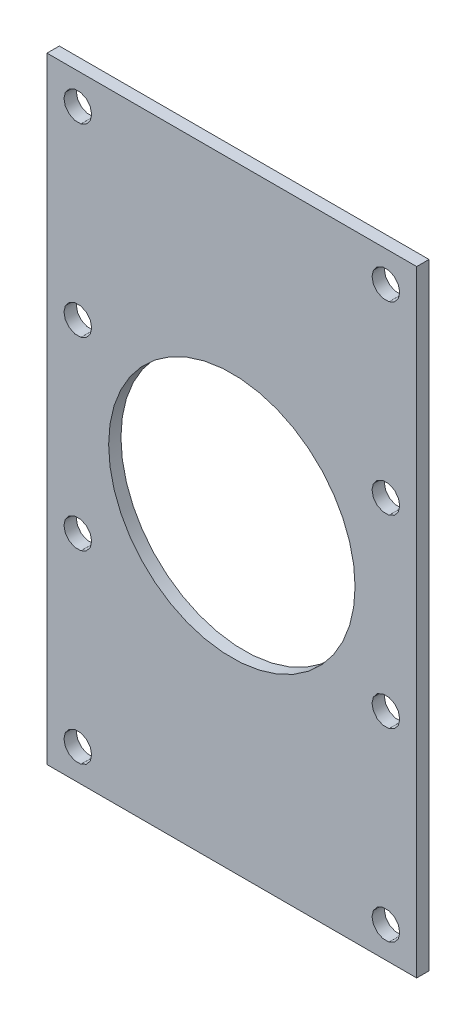
# Autodesk Inventor part: P018-Joint_carter_chapeau
Saved by Autodesk Inventor 2021.3 (Build 253353000, 353)
## iProperties
Created: 2022-05-28
Part Number: P018-Joint_carter_chapeau
Material: Polytetrafluoroethylene
Document SubType Name: Modeling
Designer: Rémi Heredero
Density: 2.02 g/cm^3
Appearance: PTFE
Author: Rémi Heredero
Autodesk Inventor part; units mm, degrees
ref_plane "YZ Plane" through (0, 0, 0) normal (1, 0, 0) x (0, 1, 0)
ref_plane "XZ Plane" through (0, 0, 0) normal (0, 1, 0) x (-1, 0, 0)
ref_plane "XY Plane" through (0, 0, 0) normal (0, 0, 1) x (1, 0, 0)
sketch "Sketch2" plane through (0, 0, 0) normal (0, 0, 1) x (1, 0, 0)
  circle A0 centre (11.25, 19.4856) radius 1.2295 projected
  circle A1 centre (11.25, -19.4856) radius 1.2295 projected
  circle A2 centre (-22.5, 0) radius 1.2295 projected
  circle A3 centre (-11.25, -19.4856) radius 1.2295 projected
  circle A4 centre (22.5, 0) radius 1.2295 projected
  circle A5 centre (-11.25, 19.4856) radius 1.2295 projected
  circle A6 centre (25, -15) radius 2.25 projected
  circle A7 centre (25, 45) radius 2.25 projected
  circle A8 centre (-25, 15) radius 2.25 projected
  circle A9 centre (-25, -45) radius 2.25 projected
  circle A10 centre (-25, -15) radius 2.25 projected
  circle A11 centre (-25, 45) radius 2.25 projected
  circle A12 centre (25, 15) radius 2.25 projected
  circle A13 centre (25, -45) radius 2.25 projected
  circle A14 centre (0, 0) radius 20 projected
  line L0 (30, -50) -> (30, 50) projected
  line L1 (-30, -50) -> (30, -50) projected
  line L2 (-30, 50) -> (-30, -50) projected
  line L3 (30, 50) -> (-30, 50) projected
extrude "Extrusion1" add sketch "Sketch2" against normal blind 2 contours A0 | A1 | A2 | A3 | A4 | A5 | L1 L2 L3 L0
body "Solid1"
